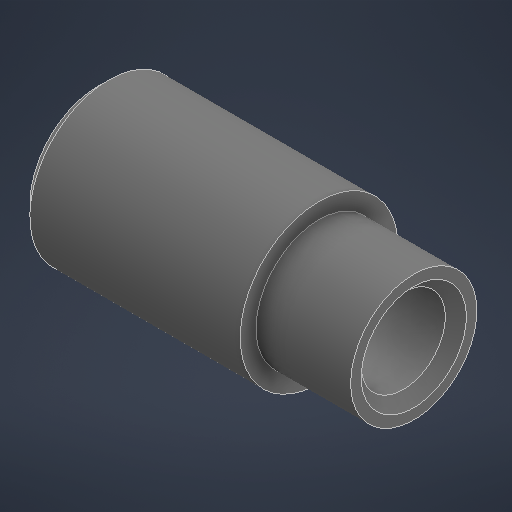
# Autodesk Inventor part: Meneteshüvely
Saved by Autodesk Inventor 2025 (Build 290162010, 162A)
## iProperties
Created: 2025-02-13
Part Number: Meneteshüvely
Material: Generic
Document SubType Name: Modeling
Designer: petruska.milan
Density: 1 g/cm^3
Appearance: Gray
Author: petruska.milan
Autodesk Inventor part; units mm, degrees
ref_plane "YZ Plane" through (0, 0, 0) normal (1, 0, 0) x (0, 1, 0)
ref_plane "XZ Plane" through (0, 0, 0) normal (0, 1, 0) x (-1, 0, 0)
ref_plane "XY Plane" through (0, 0, 0) normal (0, 0, 1) x (1, 0, 0)
sketch "Sketch1" plane through (0, 0, 0) normal (0, 0, 1) x (1, 0, 0)
  point P0 (0, 0)
sketch "Sketch2" plane through (0, 0, 0) normal (0, 0, 1) x (1, 0, 0)
  line L0 (0, 0) -> (30, 0)
  line L1 (0, 0) -> (0, 7.5)
  line L2 (0, 7.5) -> (21, 7.5)
  line L3 (30, 0) -> (30, 6)
  line L4 (30, 6) -> (21, 6)
  line L5 (21, 6) -> (21, 7.5)
  line L6 (0, 0) -> (30, 0)
  line L7 (30, 0) -> (30, 4)
  line L8 (30, 4) -> (0, 4)
  line L9 (0, 4) -> (0, 0)
  point P0 (0, 4)
  dimension "d0" = 30
  dimension "d1" = 7.5
  dimension "d2" = 21
  dimension "d3" = 6
  dimension "d4" = 4
  constraints: 20 end point, 4 perpendicular, 2 horizontal, 2 parallel, 2 vertical, 1 point on line
  measures "d0" distance of L0.start L0.end
  measures "d1" distance of L0.start L1.end
  measures "d2" distance of L1.end L2.end
  measures "d3" distance of L0.end L3.end
  measures "d4" distance of L7.end L6.end
revolve "Revolution1" add sketch "Sketch2" angle 360 about axis through (0, 0, 0) along (1, 0, 0) contours L1 L2 L5 L4 L3 L8
chamfer "Chamfer1" distance 1 angle 45 3 edges at (0, -7.5, 0) (0, -4, 0) (30, -4, 0)
body "Solid1"
